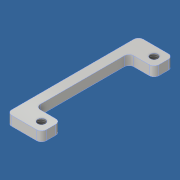
# Autodesk Inventor part: Nema23_24Mount
Saved by Autodesk Inventor 2016 SP1 (Build 200210100, 210)
## iProperties
Created: 2016-05-06
Part Number: Nema23_24Mount
Material: Aluminium 6061
Document SubType Name: Modeling
Designer: 4ndreas
Density: 2.7 g/cm^3
Appearance: Aluminium - flach
Author: 4ndreas
Autodesk Inventor part; units mm, degrees
ref_plane "YZ Plane" through (0, 0, 0) normal (1, 0, 0) x (0, 1, 0)
ref_plane "XZ Plane" through (0, 0, 0) normal (0, 1, 0) x (-1, 0, 0)
ref_plane "XY Plane" through (0, 0, 0) normal (0, 0, 1) x (1, 0, 0)
sketch "Skizze1" plane through (0, 0, 0) normal (0, 0, 1) x (1, 0, 0)
  line L0 (-2, -19.57) -> (2, -19.57)
  line L1 (2, -19.57) -> (2, 19.57)
  line L2 (2, 19.57) -> (-2, 19.57)
  line L3 (-2, 19.57) -> (-2, -19.57)
  line L4 (-2, -19.57) -> (2, 19.57) construction
  line L5 (2, -19.57) -> (-2, 19.57) construction
  line L6 (-2, 19.57) -> (10.5, 19.57)
  line L7 (12.5, 21.57) -> (12.5, 25.57)
  line L8 (10.5, 27.57) -> (0, 27.57)
  line L9 (-2, 25.57) -> (-2, 19.57)
  line L10 (-2, -19.57) -> (10.5, -19.57)
  line L11 (12.5, -21.57) -> (12.5, -25.57)
  line L12 (10.5, -27.57) -> (0, -27.57)
  line L13 (-2, -25.57) -> (-2, -19.57)
  line L14 (8.5, -23.57) -> (8.5, 23.57) construction
  circle A0 centre (8.5, -23.57) radius 4 construction
  circle A1 centre (8.5, 23.57) radius 4 construction
  circle A2 centre (8.5, 23.57) radius 2
  arc A3 (12.5, 25.57) -> (10.5, 27.57) centre (10.5, 25.57) ccw
  arc A4 (10.5, 19.57) -> (12.5, 21.57) centre (10.5, 21.57) ccw
  arc A5 (0, 27.57) -> (-2, 25.57) centre (0, 25.57) ccw
  arc A6 (-2, -25.57) -> (0, -27.57) centre (0, -25.57) ccw
  arc A7 (10.5, -27.57) -> (12.5, -25.57) centre (10.5, -25.57) ccw
  arc A8 (12.5, -21.57) -> (10.5, -19.57) centre (10.5, -21.57) ccw
  point P0 (0, 0)
  point P1 (12.5, -27.57)
  dimension "d0" = 47.14
  dimension "d1" = 6.5
  dimension "d2" = 4
  dimension "d3" = 8
  dimension "d4" = 4
  dimension "d5" = 2
  constraints: 30 end point, 18 tangent, 12 point on circle, 9 centre point, 7 parallel, 5 equal radius, 3 coincident, 3 horizontal, 3 perpendicular, 3 point on line, 2 midpoint
  measures "d0" distance of L14.start L14.end
  measures "d1" distance between parallel lines of L1 L14
  measures "d2" diameter of A2
  measures "d3" diameter of A1
  measures "d4" distance between parallel lines of L3 L1
  measures "d5" radius of A3
extrude "Extrusion1" add sketch "Skizze1" along normal blind 4 contours L3 L2 L1 L0 | L0 L10 A8 L11 A7 L12 A6 L13 | L9 A5 L8 A3 L7 A4 L6 L2 | A2
hole "Bohrung1" at (8.5, 23.57, 0) at (8.5, -23.57, 0) direction (0, 0, 1) diameter 3.242 depth 11.8 tip angle 118 thread size "M4x0.7" class "6H" standard "ANSI Metric M Profile"
fillet "Rundung1" radius 2 2 edges at (2, -19.57, 2) (2, 19.57, 2)
